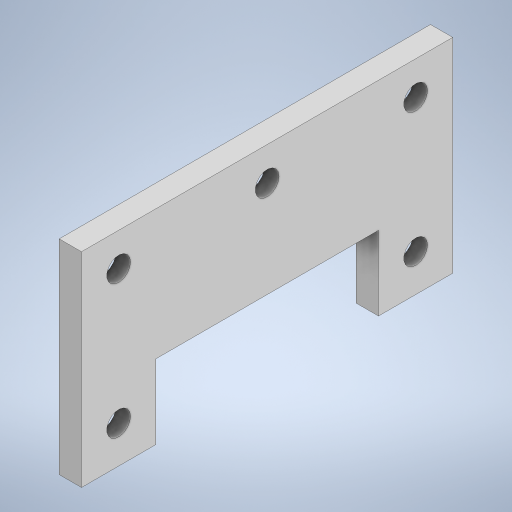
# Autodesk Inventor part: stopper
Saved by Autodesk Inventor 2023 (Build 270158000, 158)
## iProperties
Created: 2022-12-04
Part Number: stopper
Material: 一般
Document SubType Name: Modeling
Designer: RiSA
Density: 1 g/cm^3
Appearance: 既定
Author: RiSA
Autodesk Inventor part; units mm, degrees
ref_plane "YZ Plane" through (0, 0, 0) normal (1, 0, 0) x (0, 1, 0)
ref_plane "XZ Plane" through (0, 0, 0) normal (0, 1, 0) x (-1, 0, 0)
ref_plane "XY Plane" through (0, 0, 0) normal (0, 0, 1) x (1, 0, 0)
sketch "スケッチ1" plane through (0, 0, 0) normal (1, 0, 0) x (0, 1, 0)
  line L0 (-5, -25) -> (5, -25)
  line L1 (5, -25) -> (5, 25)
  line L2 (5, 25) -> (-5, 25)
  line L3 (-5, 25) -> (-5, -25)
  line L4 (-5, -25) -> (5, 25) construction
  line L5 (5, -25) -> (-5, 25) construction
  line L6 (5, 25) -> (22.5, 25)
  line L7 (22.5, 25) -> (22.5, -25)
  line L8 (22.5, -25) -> (5, -25)
  line L9 (5, -25) -> (5, 25)
  point P0 (0, 0)
  dimension "d0" = 10
  dimension "d1" = 50
  dimension "d2" = 17.5
  constraints: 20 end point, 4 parallel, 2 horizontal, 2 midpoint, 2 perpendicular
  measures "d0" distance of L2.end L1.end
  measures "d1" distance of L1.end L0.end
  measures "d2" distance of L7.end L8.end
extrude "押し出し1" add sketch "スケッチ1" along normal blind 3
sketch "スケッチ2" plane through (3, 0, 0) normal (1, 0, 0) x (0, 0, -1)
  line L0 (25, -5) -> (25, 22.5) projected
  line L1 (25, 22.5) -> (-25, 22.5) projected
  point P0 (0, 0)
  point P1 (-20, 0)
  point P2 (20, 0)
  point P3 (-20, 18)
  point P4 (0, 18)
  point P5 (20, 18)
  dimension "d5" = 40
  dimension "d6" = 5
  dimension "d7" = 4.5
  dimension "d28" = 4.5
  dimension "d29" = 4.5
  measures "d5" distance of point (20, 0) point (-20, 0)
  measures "d6" distance from line of L0 point (20, 0)
  measures "d7" distance from line of point (-20, 18) L1
  measures "d28" distance from line of L1 point (0, 18)
  measures "d29" distance from line of L1 point (20, 18)
hole "穴1" at (3, 0, 20) at (3, 0, -20) at (3, 18, 20) at (3, 18, 0) at (3, 18, -20) direction (-1, 0, 0) diameter 3.2 end through all
sketch "スケッチ3" plane through (0, 0, 0) normal (-1, 0, 0) x (0, 0, 1)
  circle A0 centre (-20, 0) radius 1.6 projected
  circle A1 centre (-20, 0) radius 3
  circle A2 centre (20, 0) radius 1.6 projected
  circle A3 centre (20, 0) radius 3
  point P0 (0, 0)
  dimension "d15" = 6
  dimension "d16" = 6
  constraints: 2 centre point, 2 coincident
  measures "d15" diameter of A1
  measures "d16" diameter of A3
extrude "押し出し2" cut sketch "スケッチ3" against normal blind 1 contours A0 | A1 | A2 | A3
sketch "スケッチ4" plane through (0, 0, 0) normal (-1, 0, 0) x (0, 0, 1)
  circle A0 centre (-20, 18) radius 1.6 projected
  circle A1 centre (-20, 18) radius 3
  circle A2 centre (0, 18) radius 1.6 projected
  circle A3 centre (0, 18) radius 3
  circle A4 centre (20, 18) radius 1.6 projected
  circle A5 centre (20, 18) radius 3
  point P0 (0, 0)
  dimension "d19" = 6
  dimension "d20" = 6
  dimension "d21" = 6
  constraints: 3 centre point, 3 coincident
  measures "d19" diameter of A1
  measures "d20" diameter of A3
  measures "d21" diameter of A5
extrude "押し出し3" cut sketch "スケッチ4" against normal blind 1 contours A0 | A1 | A3 | A4 | A5
sketch "スケッチ5" plane through (0, 0, 0) normal (-1, 0, 0) x (0, 0, 1)
  line L0 (15, 5) -> (-15, 5)
  line L1 (-15, 5) -> (-15, -5)
  line L2 (-15, -5) -> (15, -5)
  line L3 (15, -5) -> (15, 5)
  line L4 (15, 5) -> (-15, -5) construction
  line L5 (-15, 5) -> (15, -5) construction
  point P0 (0, 0)
  dimension "d24" = 30
  dimension "d25" = 10
  constraints: 12 end point, 2 midpoint, 2 parallel, 1 horizontal, 1 perpendicular
  measures "d24" distance of L2.end L1.end
  measures "d25" distance of L1.end L0.end
extrude "押し出し4" cut sketch "スケッチ5" against normal blind 3
